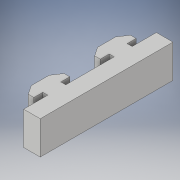
# Autodesk Inventor part: slotmountingPlate_dual_m3
Saved by Autodesk Inventor 2018 (Build 220112000, 112)
## iProperties
Created: 2020-03-14
Part Number: slotmountingPlate_dual_m3
Material: Generic
Document SubType Name: Modeling
Designer: natha
Density: 1 g/cm^3
Appearance: Default
Author: natha
Autodesk Inventor part; units mm, degrees
ref_plane "YZ Plane" through (0, 0, 0) normal (1, 0, 0) x (0, 1, 0)
ref_plane "XZ Plane" through (0, 0, 0) normal (0, 1, 0) x (-1, 0, 0)
ref_plane "XY Plane" through (0, 0, 0) normal (0, 0, 1) x (1, 0, 0)
sketch "Sketch1" plane through (0, 0, 0) normal (0, 1, 0) x (-1, 0, 0)
  line L0 (0, -5.4) -> (1.5, -5.4)
  line L1 (1.5, -5.4) -> (1.5, -8.1)
  line L2 (1.5, -8.1) -> (3.2, -8.1)
  line L3 (0, 0) -> (1.5, 0)
  line L4 (1.5, 0) -> (1.5, 2.7)
  line L5 (1.5, 2.7) -> (3.2, 2.7)
  line L6 (5, 0) -> (5, -5.4)
  line L7 (5, -5.4) -> (3.2, -8.1)
  line L8 (5, 0) -> (3.2, 2.7)
  line L9 (0, -20) -> (1.5, -20)
  line L10 (1.5, -20) -> (1.5, -17.3)
  line L11 (1.5, -17.3) -> (3.2, -17.3)
  line L12 (0, -25.4) -> (1.5, -25.4)
  line L13 (1.5, -25.4) -> (1.5, -28.1)
  line L14 (1.5, -28.1) -> (3.2, -28.1)
  line L15 (5, -20) -> (5, -25.4)
  line L16 (5, -25.4) -> (3.2, -28.1)
  line L17 (5, -20) -> (3.2, -17.3)
  line L18 (0, -5.4) -> (0, -20)
  line L19 (0, 0) -> (0, 7.3)
  line L20 (0, 7.3) -> (-5, 7.3)
  line L21 (0, -25.4) -> (0, -32.7)
  line L22 (0, -32.7) -> (-5, -32.7)
  line L23 (-5, -32.7) -> (-5, 7.3)
  dimension "d0" = 5.4
  dimension "d1" = 1.5
  dimension "d2" = 2.7
  dimension "d3" = 1.7
  dimension "d4" = 2.7
  dimension "d5" = 1.7
  dimension "d9" = 2.7
  dimension "d10" = 2.7
  dimension "d11" = 5.4
  dimension "d12" = 7.3
  dimension "d13" = 5
  dimension "d14" = 7.3
  dimension "d15" = 5
  dimension "d16" = 20
  constraints: 48 end point, 11 perpendicular, 4 vertical, 3 horizontal, 1 parallel
  measures "d0" distance of L3.start L0.start
  measures "d1" distance of L0.start L0.end
  measures "d2" distance of L0.end L1.end
  measures "d3" distance of L1.end L2.end
  measures "d4" distance of L3.end L4.end
  measures "d5" distance of L4.end L5.end
  measures "d9" distance of L9.end L10.end
  measures "d10" distance of L12.end L13.end
  measures "d11" distance between parallel lines of L12 L9
  measures "d12" distance of L3.start L19.end
  measures "d13" distance of L19.end L20.end
  measures "d14" distance of L12.start L21.end
  measures "d15" distance of L21.end L22.end
  measures "d16" distance between parallel lines of L3 L9
extrude "Extrusion1" add sketch "Sketch1" along normal blind 10
body "Solid1"
